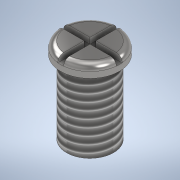
# Autodesk Inventor part: Tornillo
Saved by Autodesk Inventor 2021 (Build 250183000, 183)
## iProperties
Created: 2021-06-29
Part Number: Tornillo
Material: Acero inoxidable
Document SubType Name: Modeling
Designer: artur
Density: 8 g/cm^3
Appearance: Semipulido
Author: artur
Autodesk Inventor part; units mm, degrees
ref_plane "YZ Plane" through (0, 0, 0) normal (1, 0, 0) x (0, 1, 0)
ref_plane "XZ Plane" through (0, 0, 0) normal (0, 1, 0) x (-1, 0, 0)
ref_plane "XY Plane" through (0, 0, 0) normal (0, 0, 1) x (1, 0, 0)
sketch "Boceto1" plane through (0, 0, 0) normal (0, 0, 1) x (1, 0, 0)
  line L0 (0, 0) -> (4, 0)
  line L1 (4, 0) -> (4, 12.5)
  line L2 (4, 12.5) -> (0, 12.5)
  line L3 (0, 12.5) -> (0, 0)
  line L4 (0, 12.5) -> (5, 12.5)
  line L5 (5, 12.5) -> (5, 14.5)
  line L6 (5, 14.5) -> (0, 14.5)
  line L7 (0, 14.5) -> (0, 12.5)
  point P0 (4, 12.5)
  dimension "d0" = 4
  dimension "d1" = 12.5
  dimension "d2" = 5
  dimension "d3" = 2
  constraints: 16 end point, 4 parallel, 2 horizontal, 2 perpendicular
  measures "d0" distance of L1.end L2.end
  measures "d1" distance of L0.end L1.end
  measures "d2" distance of L5.end L6.end
  measures "d3" distance of L4.end L5.end
revolve "Revolución1" add sketch "Boceto1" angle 360 about axis through (0, 12.5, 0) along (0, -1, 0)
thread "Rosca1" size "M8x1.25" class "6g" standard "ANSI Metric M Profile" full length
sketch "Boceto2" plane through (0, 14.5, 0) normal (0, 1, 0) x (1, 0, 0)
  line L0 (-0.5, -5) -> (0.5, -5)
  line L1 (0.5, -5) -> (0.5, 5)
  line L2 (0.5, 5) -> (-0.5, 5)
  line L3 (-0.5, 5) -> (-0.5, -5)
  line L4 (5, -0.5) -> (-5, -0.5)
  line L5 (-5, -0.5) -> (-5, 0.5)
  line L6 (-5, 0.5) -> (5, 0.5)
  line L7 (5, 0.5) -> (5, -0.5)
  point P0 (0, 0)
  point P1 (0.5, 0.5)
  point P2 (0.5, -0.5)
  point P3 (-0.5, -0.5)
  point P4 (-0.5, 0.5)
  dimension "d7" = 1
  dimension "d8" = 1
  dimension "d9" = 10
  dimension "d10" = 10
  dimension "d11" = 0.5
  dimension "d12" = 0.5
  dimension "d13" = 5
  dimension "d14" = 5
  constraints: 16 end point, 4 parallel, 2 horizontal, 2 perpendicular
  measures "d7" distance of L1.end L2.end
  measures "d8" distance of L6.end L4.start
  measures "d9" distance of L0.end L1.end
  measures "d10" distance of L5.end L6.end
  measures "d11" distance from line of point (0, 0) L1
  measures "d12" distance from line of point (0, 0) L4
  measures "d13" distance from line of point (0, 0) L2
  measures "d14" distance from line of point (0, 0) L7
extrude "Extrusión1" cut sketch "Boceto2" against normal blind 1
fillet "Empalme1" radius 1 1 edges at (3.5355, 14.5, -3.5355)
fillet "Empalme2" radius 1 3 edges at (-3.5355, 14.5, -3.5355) (-3.5355, 14.5, 3.5355) (3.5355, 14.5, 3.5355)
equation "\"d8\" = d7"
equation "\"d10\" = d9"
equation "\"d11\" = 0.5 * d7"
equation "\"d12\" = 0.5 * d7"
equation "\"d13\" = 0.5 * d9"
equation "\"d14\" = 0.5 * d9"
